mount_disc (Autodesk Fusion 360 design; units mm, degrees)
part number: 2026-09-26-23-01-07-084
part number: 2026-09-26-23-23-19-979
Autodesk Fusion 360 part; units mm, degrees
note: some values were not read from the file. Set by a fixed rule: which face or edge a step refers to.
sketch "Sketch5" plane through (0, 0, 0) normal (0, 0, 1) x (1, 0, 0)
  circle A0 centre (-250, 125) radius 150
  line L0 (-250, 125) -> (-250, 250)
  circle A1 centre (-250, 250) radius 8
  circle A2 centre (-312.5, 233.2532) radius 8
  circle A3 centre (-358.2532, 187.5) radius 8
  circle A4 centre (-375, 125) radius 8
  circle A5 centre (-358.2532, 62.5) radius 8
  circle A6 centre (-312.5, 16.7468) radius 8
  circle A7 centre (-250, 0) radius 8
  circle A8 centre (-187.5, 16.7468) radius 8
  circle A9 centre (-141.7468, 62.5) radius 8
  circle A10 centre (-125, 125) radius 8
  circle A11 centre (-141.7468, 187.5) radius 8
  circle A12 centre (-187.5, 233.2532) radius 8
  dimension "d20" = 300
  dimension "d21" = 16
  dimension "d23" = 360
  constraint coincident A0.centre L0.start
  constraint vertical L0
  constraint coincident L0.end A1.centre
  measures "d20" diameter of A0
  measures "d21" diameter of A1
extrude "Extrude4" add sketch "Sketch5" along normal blind 5 makes body 1
sketch "Sketch6" plane through (0, 0, 5) normal (0, 0, 1) x (-1, 0, 0)
  circle A0 centre (125, -125) radius 8
  circle A1 centre (187.5, -233.2532) radius 8
  circle A2 centre (250, -125) radius 150
  circle A3 centre (250, -250) radius 8
  circle A4 centre (375, -125) radius 8
  circle A5 centre (312.5, -233.2532) radius 8
  circle A6 centre (250, 0) radius 8
  circle A7 centre (141.7468, -62.5) radius 8
  circle A8 centre (358.2532, -187.5) radius 8
  circle A9 centre (141.7468, -187.5) radius 8
  circle A10 centre (312.5, -16.7468) radius 8
  circle A11 centre (358.2532, -62.5) radius 8
  circle A12 centre (187.5, -16.7468) radius 8
  arc A13 (187.5, -233.2532) -> (250, -250) centre (260.797, -84.705) ccw
  circle A14 centre (217.9243, -244.708) radius 8
  circle A15 centre (369.708, -157.0757) radius 8
  circle A16 centre (282.0757, -5.292) radius 8
  circle A17 centre (130.292, -92.9243) radius 8
  dimension "d26" = 16
  dimension "d28" = 360
  constraint coincident A1.centre A13.start
  constraint coincident A3.centre A13.end
  constraint midpoint A13 A14.centre
  measures "d26" diameter of A14
extrude "Extrude5" add sketch "Sketch6" along normal blind 10 contours A13 A14 | A13 A14 | A15 | A16 | A17 bodies 1
sketch "Sketch7" plane through (0, 0, 15) normal (0, 0, 1) x (-1, 0, 0)
  circle A0 centre (282.0757, -5.292) radius 8
  circle A1 centre (282.0757, -5.292) radius 2
  dimension "d31" = 4
  constraint concentric A0 A1
  measures "d31" diameter of A1
sketch "Sketch8" plane through (0, 0, 0) normal (0, 0, 1) x (1, 0, 0)
sketch "Sketch9" plane through (0, 0, 15) normal (0, 0, 1) x (-1, 0, 0)
  circle A0 centre (130.292, -92.9243) radius 8
  circle A1 centre (130.292, -92.9243) radius 2
  dimension "d32" = 4
  constraint concentric A0 A1
  measures "d32" diameter of A1
sketch "Sketch10" plane through (0, 0, 15) normal (0, 0, 1) x (-1, 0, 0)
  circle A0 centre (217.9243, -244.708) radius 8
  circle A1 centre (218, -245) radius 2
  dimension "d33" = 4
  measures "d33" diameter of A1
sketch "Sketch11" plane through (0, 0, 15) normal (0, 0, 1) x (-1, 0, 0)
  circle A0 centre (369.708, -157.0757) radius 8
  circle A1 centre (369.708, -157.0757) radius 2
  dimension "d34" = 4
  constraint concentric A0 A1
  measures "d34" diameter of A1
extrude "Extrude6" cut sketch "Sketch11" sketch "Sketch10" sketch "Sketch9" sketch "Sketch7" against normal blind 5 contours A1 of sketch 2 contours A1 of sketch 3 contours A1 of sketch 4 contours A1 bodies 1
thread "Thread2" "ISO Metric profile 4.0 M4x0.7 M4x0.7 6H" major diameter 4.1095 minor diameter 3.332 pitch 0.7 angle 60 resizes the face on face at (-282.9881, 3.5123, 11.6667) on face at (-131.6154, 91.4248, 11.6667) on face at (-219.9382, 244.5065, 11.6667) on face at (-371.4644, 158.0322, 11.6667) on bodies 1
copy_body "Body->Comp1" bodies 1 removing the originals makes body 2 in component "Component"
sketch "Sketch1" plane through (0, 0, 0) normal (0, 0, 1) x (1, 0, 0)
sketch "Sketch2" plane through (0, 0, 0) normal (1, 0, 0) x (0, 1, 0)
  circle A0 centre (-250, 250) radius 150
  line L0 (-250, 250) -> (-250, 375)
  circle A1 centre (-250, 375) radius 8
  circle A2 centre (-312.5, 358.2532) radius 8
  circle A3 centre (-358.2532, 312.5) radius 8
  circle A4 centre (-375, 250) radius 8
  circle A5 centre (-358.2532, 187.5) radius 8
  circle A6 centre (-312.5, 141.7468) radius 8
  circle A7 centre (-250, 125) radius 8
  circle A8 centre (-187.5, 141.7468) radius 8
  circle A9 centre (-141.7468, 187.5) radius 8
  circle A10 centre (-125, 250) radius 8
  circle A11 centre (-141.7468, 312.5) radius 8
  circle A12 centre (-187.5, 358.2532) radius 8
  line L1 (-250, 375) -> (-187.5, 358.2532)
  line L2 (-250, 375) -> (-218.75, 366.6266)
  circle A13 centre (-220.2756, 367.0354) radius 8
  dimension "d1" = 300
  dimension "d2" = 16
  dimension "d4" = 360
  dimension "d5" = 16
  constraint coincident A0.centre L0.start
  constraint vertical L0
  constraint coincident L0.end A1.centre
  constraint coincident A12.centre L1.end
  constraint midpoint L1 L2.end
  constraint coincident L1 A13.centre
  measures "d1" diameter of A0
  measures "d2" diameter of A1
  measures "d5" diameter of A13
extrude "Extrude1" [rolled back] along distance 5 taper angle 0
sketch "Sketch3" plane through (5, 0, 0) normal (1, 0, 0) x (0, 1, 0)
  circle A0 centre (-141.7468, 187.5) radius 8
  circle A1 centre (-250, 125) radius 8
  circle A2 centre (-250, 250) radius 150
  circle A3 centre (-187.5, 358.2532) radius 8
  circle A4 centre (-250, 375) radius 8
  circle A5 centre (-358.2532, 312.5) radius 8
  circle A6 centre (-312.5, 358.2532) radius 8
  circle A7 centre (-375, 250) radius 8
  circle A8 centre (-358.2532, 187.5) radius 8
  circle A9 centre (-187.5, 141.7468) radius 8
  circle A10 centre (-312.5, 141.7468) radius 8
  circle A11 centre (-141.7468, 312.5) radius 8
  circle A12 centre (-125, 250) radius 8
  line L0 (-250, 375) -> (-187.5, 358.2532)
  circle A13 centre (-218.75, 366.6266) radius 8
  circle A14 centre (-366.6266, 281.25) radius 8
  circle A15 centre (-281.25, 133.3734) radius 8
  circle A16 centre (-133.3734, 218.75) radius 8
  dimension "d8" = 16
  dimension "d10" = 360
  constraint coincident A4.centre L0.start
  constraint coincident A3.centre L0.end
  constraint midpoint L0 A13.centre
  measures "d8" diameter of A13
extrude "Extrude2" [rolled back] along distance 10 taper angle 0
sketch "Sketch4" plane through (15, 0, 0) normal (1, 0, 0) x (0, 1, 0)
  circle A0 centre (-281.25, 133.3734) radius 8
  circle A1 centre (-281.25, 133.3734) radius 2
  circle A2 centre (-367, 281) radius 2
  circle A3 centre (-218.6865, 366.4726) radius 2
  circle A4 centre (-133.5814, 218.3266) radius 2
  dimension "d13" = 4
  dimension "d14" = 4
  dimension "d15" = 4
  constraint concentric A0 A1
  measures "d13" diameter of A1
  measures "d14" diameter of A3
  measures "d15" diameter of A4
extrude "Extrude3" [rolled back] along distance -5 taper angle 0
thread "Thread1" [rolled back] thread offset 0 thread length 10
component "Component" placed x (1, 0, 0) y (0, 1, 0) z (0, 0, 1) at (0, 0, 0)
